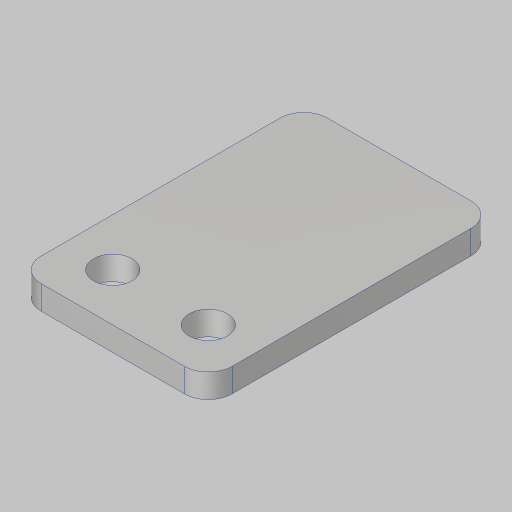
# Autodesk Inventor part: EL2-035
Saved by Autodesk Inventor 2023.5 (Build 275446000, 446)
## iProperties
Created: 2025-01-21
Part Number: EL2-035
Material: Aluminum 6061
Document SubType Name: Modeling
Designer: slick
Density: 2.7 g/cm^3
Appearance: Aluminum - Flat
Author: slick
Autodesk Inventor part; units mm, degrees
ref_plane "YZ Plane" through (0, 0, 0) normal (1, 0, 0) x (0, 1, 0)
ref_plane "XZ Plane" through (0, 0, 0) normal (0, 1, 0) x (-1, 0, 0)
ref_plane "XY Plane" through (0, 0, 0) normal (0, 0, 1) x (1, 0, 0)
sketch "Sketch1" plane through (0, 0, 0) normal (0, 1, 0) x (-1, 0, 0)
  line L0 (8.89, 0) -> (-8.89, 0) construction
  line L1 (8.89, 1.5875) -> (-8.89, 1.5875)
  line L2 (-8.89, -1.5875) -> (8.89, -1.5875)
  arc A0 (8.89, -1.5875) -> (8.89, 1.5875) centre (8.89, 0) ccw
  arc A1 (-8.89, 1.5875) -> (-8.89, -1.5875) centre (-8.89, 0) ccw
  line L3 (8.89, -5.0038) -> (-8.89, -5.0038) construction
  line L4 (8.89, -3.4163) -> (-8.89, -3.4163)
  line L5 (-8.89, -6.5913) -> (8.89, -6.5913)
  arc A2 (8.89, -6.5913) -> (8.89, -3.4163) centre (8.89, -5.0038) ccw
  arc A3 (-8.89, -3.4163) -> (-8.89, -6.5913) centre (-8.89, -5.0038) ccw
  line L6 (8.89, -10.0076) -> (-8.89, -10.0076) construction
  line L7 (8.89, -8.4201) -> (-8.89, -8.4201)
  line L8 (-8.89, -11.5951) -> (8.89, -11.5951)
  arc A4 (8.89, -11.5951) -> (8.89, -8.4201) centre (8.89, -10.0076) ccw
  arc A5 (-8.89, -8.4201) -> (-8.89, -11.5951) centre (-8.89, -10.0076) ccw
  line L9 (12.7, 20.1549) -> (-12.7, 20.1549)
  line L10 (-12.7, 20.1549) -> (-12.7, -17.9451)
  line L11 (-12.7, -17.9451) -> (12.7, -17.9451)
  line L12 (12.7, -17.9451) -> (12.7, 20.1549)
  line L13 (6.35, 13.8049) -> (-6.35, 13.8049) construction
  line L14 (-8.89, -16.5989) -> (8.89, -16.5989)
  arc A6 (8.89, -16.5989) -> (8.89, -13.4239) centre (8.89, -15.0114) ccw
  line L15 (8.89, -13.4239) -> (-8.89, -13.4239)
  line L16 (8.89, -15.0114) -> (-8.89, -15.0114) construction
  arc A7 (-8.89, -13.4239) -> (-8.89, -16.5989) centre (-8.89, -15.0114) ccw
  point P0 (0, 0)
  point P1 (0, -5.0038)
  point P2 (0, -10.0076)
  point P3 (10.4775, -5.0038)
  point P4 (10.4775, 0)
  point P5 (10.4775, -10.0076)
  point P6 (0, -17.9451)
  point P7 (0, -11.5951)
  point P8 (0, 13.8049)
  point P9 (0, 20.1549)
  point P10 (0, -16.5989)
  point P11 (10.4775, -15.0114)
  dimension "d1" = 17.78
  dimension "d3" = 3.175
  dimension "d4" = 5.0038
  dimension "d5" = 5.0038
  dimension "d8" = 25.4
  dimension "d9" = 38.1
  dimension "d10" = 6.35
  dimension "d11" = 12.7
  dimension "d12" = 6.35
  dimension "d25" = 5.0038
  constraints: 42 end point, 19 point on circle, 12 tangent, 9 parallel, 8 centre point, 7 midpoint, 4 vertical alignment, 3 horizontal, 2 equal radius, 1 horizontal alignment, 1 perpendicular, 1 vertical, 13 other
  measures "d1" distance of L1.start L1.end
  measures "d3" distance between parallel lines of L2 L1
  measures "d4" distance of point (10.477, -5.004) point (10.477, 0)
  measures "d5" distance of point (10.477, -10.008) point (10.477, -5.004)
  measures "d8" distance of L10.end L11.end
  measures "d9" distance of L11.end L9.start
  measures "d10" distance of point (0, -11.595) point (0, -17.945)
  measures "d11" distance of L13.start L13.end
  measures "d12" distance from line of L9 L13.start
  measures "d25" distance of L8.start L14.start
extrude "Extrusion1" add sketch "Sketch1" along normal blind 3.175 contours A0 L2 A1 L1 | A2 L5 A3 L4 | A4 L8 A5 L7 | L12 L11 L10 L9 | A7 L15 A6 L14
hole "Hole1" at (-6.35, 0, 13.8049) at (6.35, 0, 13.8049) direction (0, 1, 0) diameter 5.1054 end through all clearance for "Flat Head Machine Screw (82)" size "#10" standard "Ansi Unified Screw Threads"
fillet "Fillet1" radius 3.175 4 edges at (-12.7, 1.5875, -17.9451) (12.7, 1.5875, -17.9451) (12.7, 1.5875, 20.1549) (-12.7, 1.5875, 20.1549)
equation "\"d5\" = d4"
body "Solid1"
